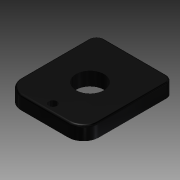
# Autodesk Inventor part: Durometer_Base
Saved by Autodesk Inventor 2015 (Build 190159000, 159)
## iProperties
Created: 2014-12-16
Part Number: Durometer_Base
Material: Generic
Document SubType Name: Modeling
Designer: amarschn
Density: 1 g/cm^3
Appearance: Glossy - Black
Author: amarschn
Autodesk Inventor part; units mm, degrees
ref_plane "YZ Plane" through (0, 0, 0) normal (1, 0, 0) x (0, 1, 0)
ref_plane "XZ Plane" through (0, 0, 0) normal (0, 1, 0) x (-1, 0, 0)
ref_plane "XY Plane" through (0, 0, 0) normal (0, 0, 1) x (1, 0, 0)
sketch "Sketch1" plane through (0, 0, 0) normal (0, 1, 0) x (-1, 0, 0)
  line L0 (-61.2, -88.9) -> (61.2, -88.9)
  line L1 (76.2, -73.9) -> (76.2, 58.9)
  line L2 (46.2, 88.9) -> (-46.2, 88.9)
  line L3 (-76.2, 58.9) -> (-76.2, -73.9)
  line L4 (-76.2, -88.9) -> (76.2, 88.9) construction
  line L5 (76.2, -88.9) -> (-76.2, 88.9) construction
  arc A0 (76.2, 58.9) -> (46.2, 88.9) centre (46.2, 58.9) ccw
  arc A1 (-46.2, 88.9) -> (-76.2, 58.9) centre (-46.2, 58.9) ccw
  arc A2 (61.2, -88.9) -> (76.2, -73.9) centre (61.2, -73.9) ccw
  arc A3 (-76.2, -73.9) -> (-61.2, -88.9) centre (-61.2, -73.9) ccw
  circle A4 centre (0, 73.025) radius 7.9375
  circle A5 centre (0, 0) radius 27.5
  dimension "d0" = 177.8
  dimension "d1" = 152.4
  dimension "d2" = 30
  dimension "d3" = 15
  dimension "d4" = 15.875
  dimension "d5" = 15.875
  dimension "d9" = 55
  constraints: 12 end point, 8 point on circle, 8 point on line, 8 tangent, 6 centre point, 2 equal radius, 2 midpoint, 2 parallel, 1 coincident, 1 horizontal, 1 perpendicular
  measures "d0" distance of L5.start L4.end
  measures "d1" distance of L4.end L5.end
  measures "d2" radius of A0
  measures "d3" radius of A2
  measures "d4" distance from line of L2 A4.centre
  measures "d5" diameter of A4
  measures "d9" diameter of A5
extrude "Extrusion1" add sketch "Sketch1" along normal blind 26.75
fillet "Fillet1" radius 4 8 edges at (71.8066, 26.75, -84.5066) (0, 26.75, -88.9) (-71.8066, 26.75, -84.5066) (-76.2, 26.75, -7.5) (-67.4132, 26.75, 80.1132) (0, 26.75, 88.9) (67.4132, 26.75, 80.1132) (76.2, 26.75, -7.5)
body "Solid1"
